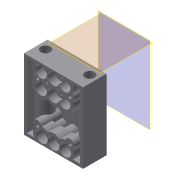
# Autodesk Inventor part: 20_Base_STORMchip_doublesided_railsystem_Laser
Saved by Autodesk Inventor 2019 (Build 230136000, 136)
## iProperties
Created: 2018-10-09
Part Number: 20_Base_STORMchip_doublesided_railsystem_Laser
Material: Generic
Document SubType Name: Modeling
Designer: diederichbenedict
Density: 1 g/cm^3
Appearance: Default
Author: diederichbenedict
Autodesk Inventor part; units mm, degrees
ref_plane "YZ Plane" through (0, 0, 0) normal (1, 0, 0) x (0, 1, 0)
ref_plane "XZ Plane" through (0, 0, 0) normal (0, 1, 0) x (-1, 0, 0)
ref_plane "XY Plane" through (0, 0, 0) normal (0, 0, 1) x (1, 0, 0)
ref_plane "Work Plane1" through (32, 0, -32) normal (0, 0, -1) x (-1, 0, 0)
ref_plane "Work Plane2" through (16, 48, -16) normal (0, 1, 0) x (0, 0, 1)
sketch "Sketch1" plane through (16, 48, -16) normal (0, 1, 0) x (0, 0, 1)
  circle A0 centre (0, 0) radius 6 projected
  line L0 (16, 16) -> (-16, 16) projected
  line L1 (-16, 16) -> (-16, -16) projected
  line L2 (-16, -16) -> (16, -16) projected
  line L3 (16, -16) -> (16, 16) projected
  line L4 (-10.5141, -20.066) -> (25.3435, -20.066) construction
  line L5 (25.3435, -20.066) -> (27.4807, -17.9288) construction
  line L6 (27.4807, -17.9288) -> (27.4807, 17.9288) construction
  line L7 (27.4807, 17.9288) -> (25.3435, 20.066) construction
  line L8 (25.3435, 20.066) -> (-10.5141, 20.066) construction
  line L9 (-10.5141, 20.066) -> (-12.6513, 17.9288) construction
  line L10 (-12.6513, 17.9288) -> (-12.6513, -17.9288) construction
  line L11 (-12.6513, -17.9288) -> (-10.5141, -20.066) construction
  circle A1 centre (22.4147, 15) radius 3.2639 construction
  circle A2 centre (22.4147, -15) radius 3.2639 construction
  circle A3 centre (-7.5852, 15) radius 3.2639 construction
  circle A4 centre (-7.5852, -15) radius 3.2639 construction
  circle A5 centre (7.4147, 0) radius 13.3985 construction
  line L12 (16, -20.066) -> (32.8642, -20.066) construction
  line L13 (32.8642, -20.066) -> (32.8642, 20.066) construction
  line L14 (32.8642, 20.066) -> (16, 20.066) construction
  line L15 (16, 20.066) -> (16, -20.066) construction
  line L16 (16, -20.066) -> (32, -20.066)
  line L17 (32, -20.066) -> (32, 20.066)
  line L18 (32, 20.066) -> (16, 20.066)
  line L19 (16, 20.066) -> (16, -20.066)
  line L20 (25.3435, 20.066) -> (-10.5141, 20.066) projected
  circle A6 centre (22.4147, -15) radius 3.25
  circle A7 centre (22.4147, 15) radius 3.25
  point P0 (24, 20.066)
  dimension "d0" = 16
  dimension "d2" = 6.5
  dimension "d3" = 6.5
  constraints: 16 end point, 4 parallel, 3 point on line, 2 centre point, 2 coincident, 2 horizontal, 2 perpendicular, 1 midpoint
  measures "d0" distance of L18.end L17.end
  measures "d2" diameter of A6
  measures "d3" diameter of A7
ref_plane "Work Plane3" through (0, 0, -32) normal (0, -1, 0) x (1, 0, 0)
extrude "Extrusion1" add sketch "Sketch1" against normal up to surface (48 mm away) contours L19 L18 L17 L16 L3
sketch "Sketch2" plane through (-4.066, 48, 16) normal (0, 0, 1) x (1, 0, 0)
  circle A0 centre (12.066, -43) radius 1 projected
  line L0 (40.132, -48) -> (0, -48) projected
  line L1 (0, 0) -> (0, -48) projected
  line L2 (40.132, 0) -> (0, 0) projected
  line L3 (40.132, 0) -> (40.132, -48) projected
  circle A1 centre (20.066, -43) radius 1 projected
  circle A2 centre (28.066, -43) radius 1 projected
  circle A3 centre (27.566, -15) radius 1 projected
  circle A4 centre (20.066, -15) radius 1 projected
  circle A5 centre (11.566, -15) radius 1.0474 projected
  circle A6 centre (27.566, -5) radius 1 projected
  circle A7 centre (20.066, -5) radius 1 projected
  circle A8 centre (11.566, -5) radius 1 projected
  point P0 (4.066, -48)
hole "Hole1" at (24, 5, 16) at (16, 5, 16) at (8, 5, 16) at (7.5, 33, 16) at (16, 33, 16) at (23.5, 33, 16) at (23.5, 43, 16) at (16, 43, 16) at (7.5, 43, 16) direction (0, 0, -1) diameter 4 end through all counterbore diameter 8 counterbore depth 5
sketch "Sketch4" plane through (-4.066, 48, 16) normal (0, 0, 1) x (1, 0, 0)
  line L0 (2.0561, 116.1804) -> (2.0561, -43.8196)
  line L1 (8.0759, 116.1804) -> (8.0759, -43.8196)
  line L2 (32.0561, 115.9357) -> (32.0561, -44.0643)
  line L3 (38.0759, 115.9357) -> (38.0759, -44.0643)
  circle A0 centre (31.0561, -10) radius 1.25
  line L4 (0, 0) -> (40.132, 0) projected
  circle A1 centre (31.0561, -38) radius 1.25
  line L5 (0, -48) -> (40.132, -48) projected
  circle A2 centre (9.0759, -38) radius 1.25
  circle A3 centre (9.0759, -10) radius 1.25
  point P0 (4.066, -48)
  dimension "d13" = 2.5
  dimension "d15" = 1
  dimension "d16" = 10
  dimension "d17" = 2.5
  dimension "d18" = 10
  dimension "d19" = 2.5
  dimension "d20" = 1
  dimension "d21" = 2.5
  constraints: 8 end point, 4 centre point, 4 vertical, 8 other
  measures "d13" diameter of A0
  measures "d15" distance from line of L2 A0.centre
  measures "d16" distance from line of A0.centre L4
  measures "d17" diameter of A1
  measures "d18" distance from line of A1.centre L5
  measures "d19" diameter of A2
  measures "d20" distance from line of L1 A2.centre
  measures "d21" diameter of A3
extrude "Extrusion2" cut sketch "Sketch4" against normal through all
shell "Shell1" thickness 2 removed faces 1 at (33.2009, 26.8389, 16)
body "Solid1"
